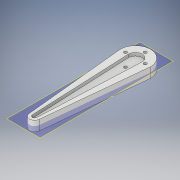
# Autodesk Inventor part: Delta_Arm
Saved by Autodesk Inventor 2019 (Build 230136000, 136)
## iProperties
Created: 2019-07-06
Part Number: Delta_Arm
Material: ABS Plastic
Document SubType Name: Modeling
Designer: Jorian Brusind
Density: 1.06 g/cm^3
Appearance: Smooth - White
Author: Jorian Brusind
Autodesk Inventor part; units mm, degrees
ref_plane "YZ Plane" through (0, 0, 0) normal (1, 0, 0) x (0, 1, 0)
ref_plane "XZ Plane" through (0, 0, 0) normal (0, 1, 0) x (-1, 0, 0)
ref_plane "XY Plane" through (0, 0, 0) normal (0, 0, 1) x (1, 0, 0)
sketch "Sketch1" plane through (0, 0, 0) normal (0, 1, 0) x (-1, 0, 0)
  circle A0 centre (0, 0) radius 5
  line L0 (0, 0) -> (0, -100)
  circle A1 centre (0, -100) radius 15
  line L1 (5, 0) -> (15, -100)
  line L2 (-5, 0) -> (-15, -100)
  dimension "d0" = 10
  dimension "d1" = 100
  dimension "d2" = 30
  dimension "d3" = 100
  dimension "d4" = 5.711
  dimension "d5" = 5.711
  dimension "d6" = 100
  constraints: 6 end point, 4 point on circle, 2 centre point, 2 coincident, 1 vertical
  measures "d0" diameter of A0
  measures "d1" distance of L0.start L0.end
  measures "d2" diameter of A1
  measures "d3" vertical distance of L1.start L1.end
  measures "d4" angle of L0 L1
  measures "d5" angle of L0 L2
  measures "d6" vertical distance of L2.start L2.end
extrude "Extrusion1" add sketch "Sketch1" along normal blind 10 contours A0 | L1 A1 L0 A0 | A0 L0 A1 L2 | L1 A1 L2
sketch "Sketch2" plane through (0, 10, 0) normal (0, 1, 0) x (1, 0, 0)
  circle A0 centre (0, 0) radius 2.25
  dimension "d9" = 4.5
  constraints: 1 centre point, 1 coincident
  measures "d9" diameter of A0
extrude "Extrusion2" cut sketch "Sketch2" against normal blind 10
sketch "Sketch3" plane through (0, 10, 0) normal (0, 1, 0) x (1, 0, 0)
  arc A0 (15, 100) -> (-15, 100) centre (0, 100) ccw projected
  circle A1 centre (0, 0) radius 2.25 projected
  line L0 (0, 0) -> (2.25, 0) construction
  line L1 (0, 100) -> (-6.75, 100)
  line L2 (0, 100) -> (6.75, 100) construction
  line L3 (0, 100) -> (6.75, 100)
  line L4 (6.75, 100) -> (2.25, 0)
  line L5 (-2.25, 0) -> (-6.75, 100)
  line L6 (0, 0) -> (-2.25, 0)
  line L7 (0, 0) -> (2.25, 0)
  arc A2 (6.75, 100) -> (-6.75, 100) centre (0, 100) ccw
  dimension "d15" = 2.25
  dimension "d16" = 6.75
  dimension "d17" = 180
  dimension "d18" = 2.25
  constraints: 16 end point, 4 horizontal, 3 collinear, 2 point on circle, 1 centre point, 1 coincident
  measures "d15" distance of L6.start L5.start
  measures "d16" distance of L1.start L1.end
  measures "d17" angle of L1 L2
  measures "d18" distance of L0.start L0.end
extrude "Extrusion3" cut sketch "Sketch3" against normal blind 3 contours L7 L6 A1 | A1 L5 L1 L3 L4 | L3 L1 A2 picked at (-1.4782, 0.1795)
sketch "Sketch4" plane through (0, 10, 0) normal (0, 1, 0) x (1, 0, 0)
  arc A0 (6.75, 100) -> (-6.75, 100) centre (0, 100) ccw projected
  line L0 (0, 100) -> (-9.779, 100)
  circle A1 centre (-9.779, 100) radius 1.5
  circle A2 centre (0, 109.779) radius 1.5
  circle A3 centre (9.779, 100) radius 1.5
  circle A4 centre (0, 90.221) radius 1.5
  point P0 (0, 0)
  dimension "d21" = 9.779
  dimension "d22" = 3
  dimension "d25" = 360
  constraints: 4 centre point, 2 end point, 1 coincident, 1 horizontal, 9 other
  measures "d21" distance of L0.start L0.end
  measures "d22" diameter of A1
extrude "Extrusion4" cut sketch "Sketch4" against normal blind 10
sketch "Sketch6" plane through (0, 0, 0) normal (0, -1, 0) x (1, 0, 0)
  arc A0 (-3.2257, -110.762) -> (3.2257, -110.762) centre (0, -109.779) ccw
  arc A1 (-9.0202, -104.6756) -> (-4.6756, -109.0202) centre (0, -100) ccw
  circle A2 centre (-9.779, 0) radius 1.5
  circle A3 centre (0, 9.779) radius 1.5
  arc A4 (-9.0202, -104.6756) -> (-10.762, -103.2257) centre (-11.6135, -106.0199) ccw
  arc A5 (-10.762, -96.7743) -> (-10.762, -103.2257) centre (-9.779, -100) ccw
  arc A6 (-3.2257, -110.762) -> (-4.6756, -109.0202) centre (-6.0199, -111.6135) ccw
  arc A7 (4.6756, -109.0202) -> (9.0202, -104.6756) centre (0, -100) ccw
  arc A8 (4.6756, -109.0202) -> (3.2257, -110.762) centre (6.0199, -111.6135) ccw
  arc A9 (10.762, -103.2257) -> (10.762, -96.7743) centre (9.779, -100) ccw
  arc A10 (10.762, -103.2257) -> (9.0202, -104.6756) centre (11.6135, -106.0199) ccw
  arc A11 (9.0202, -95.3244) -> (4.6756, -90.9798) centre (0, -100) ccw
  arc A12 (9.0202, -95.3244) -> (10.762, -96.7743) centre (11.6135, -93.9801) ccw
  arc A13 (3.2257, -89.238) -> (4.6756, -90.9798) centre (6.0199, -88.3865) ccw
  arc A14 (3.2257, -89.238) -> (-3.2257, -89.238) centre (0, -90.221) ccw
  arc A15 (-4.6756, -90.9798) -> (-9.0202, -95.3244) centre (0, -100) ccw
  arc A16 (-4.6756, -90.9798) -> (-3.2257, -89.238) centre (-6.0199, -88.3865) ccw
  arc A17 (-10.762, -96.7743) -> (-9.0202, -95.3244) centre (-11.6135, -93.9801) ccw
  circle A18 centre (0, -109.779) radius 1.5 projected
  dimension "d32" = 9.779
  constraints: 32 point on circle, 18 centre point
  measures "d32" distance of A18.centre A1.centre
extrude "Extrusion5" cut sketch "Sketch6" against normal blind 3 contours A6 A1 A4 A5 A17 A15 A16 A14 A13 A11 A12 A9 A10 A7 A8 A0
ref_plane "Work Plane1" through (0, 5, 0) normal (0, -1, 0) x (1, 0, 0)
mirror "Mirror1" about plane through (0, 5, 0) normal (0, -1, 0) of "Extrusion3"
body "Solid1"
